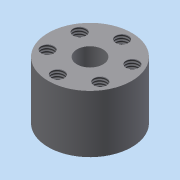
# Autodesk Inventor part: moyeux_expansible
Saved by Autodesk Inventor 2016 (Build 200138000, 138)
## iProperties
Created: 2016-12-04
Part Number: moyeux_expansible
Material: Generic
Document SubType Name: Modeling
Designer: Aegir
Density: 1 g/cm^3
Appearance: Default
Author: Aegir
Autodesk Inventor part; units mm, degrees
ref_plane "YZ Plane" through (0, 0, 0) normal (1, 0, 0) x (0, 1, 0)
ref_plane "XZ Plane" through (0, 0, 0) normal (0, 1, 0) x (-1, 0, 0)
ref_plane "XY Plane" through (0, 0, 0) normal (0, 0, 1) x (1, 0, 0)
sketch "Esquisse1" plane through (0, 0, 0) normal (0, 0, 1) x (1, 0, 0)
  circle A0 centre (0, 0) radius 8
  circle A1 centre (0, 0) radius 2.5
  point P0 (0.1533, 6)
  point P1 (-5.1195, 3.1328)
  point P2 (-5.2728, -2.8672)
  point P3 (-0.1533, -6)
  point P4 (5.1195, -3.1328)
  point P5 (5.2728, 2.8672)
  dimension "d0" = 5
  dimension "d1" = 16
  dimension "d2" = 6
  dimension "d5" = 360
  constraints: 2 centre point, 2 coincident, 7 other
  measures "d0" diameter of A1
  measures "d1" diameter of A0
  measures "d2" vertical distance of A0.centre point (0.153, 6)
extrude "Extrusion1" add sketch "Esquisse1" against normal blind 11
sketch "Esquisse2" plane through (0, 0, 0) normal (0, 0, 1) x (1, 0, 0)
  circle A0 centre (0, 0) radius 8 projected
  point P0 (0.16, 6)
  point P1 (-5.1161, 3.1386)
  point P2 (-5.2762, -2.8614)
  point P3 (-0.16, -6)
  point P4 (5.1161, -3.1386)
  point P5 (5.2762, 2.8614)
  dimension "d9" = 6
  dimension "d12" = 360
  constraints: 2 coincident, 11 other
  measures "d9" vertical distance of A0.centre point (0.16, 6)
hole "Perçage1" at (0.16, 6, 0) at (-5.1161, 3.1386, 0) at (-5.2762, -2.8614, 0) at (-0.16, -6, 0) at (5.1161, -3.1386, 0) at (5.2762, 2.8614, 0) direction (0, 0, -1) diameter 2.459 depth 8.8 tip angle 118 thread size "M3x0.5" class "6H" standard "ISO Metric profile"
